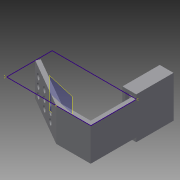
# Autodesk Inventor part: PiCamWalkerMount
Saved by Autodesk Inventor 2015 (Build 190159000, 159)
## iProperties
Created: 2016-04-28
Part Number: PiCamWalkerMount
Material: Generic
Document SubType Name: Modeling
Designer: Hatch
Density: 1 g/cm^3
Appearance: Default
Author: Hatch
Autodesk Inventor part; units mm, degrees
ref_plane "YZ Plane" through (0, 0, 0) normal (1, 0, 0) x (0, 1, 0)
ref_plane "XZ Plane" through (0, 0, 0) normal (0, 1, 0) x (-1, 0, 0)
ref_plane "XY Plane" through (0, 0, 0) normal (0, 0, 1) x (1, 0, 0)
sketch "Sketch1" plane through (0, 0, 0) normal (0, 1, 0) x (-1, 0, 0)
  line L0 (0, 0) -> (36, 0)
  line L1 (36, 0) -> (36, -24)
  line L2 (36, -24) -> (0, -24)
  line L3 (0, -24) -> (0, 0)
  dimension "d0" = 36
  dimension "d1" = 24
  constraints: 8 end point, 2 parallel, 1 horizontal, 1 perpendicular
  measures "d0" distance of L1.end L2.end
  measures "d1" distance of L0.end L1.end
extrude "Extrusion1" add sketch "Sketch1" along normal blind 3
sketch "Sketch2" plane through (0, 3, 0) normal (0, 1, 0) x (1, 0, 0)
  circle A0 centre (-6, 12) radius 2.125
  point P0 (0, 0)
  dimension "d4" = 4.25
  constraints: 1 centre point
  measures "d4" diameter of A0
extrude "Extrusion2" cut sketch "Sketch2" against normal through all
pattern_linear "Rectangular Pattern1" count 3 spacing 12 along (-1, 0, 0) count 3 spacing 6 along (0, 0, 1) of "Extrusion2" second direction both ways yes
sketch "Sketch3" plane through (0, 0, 0) normal (1, 0, 0) x (0, 0, -1)
  line L0 (0, 0) -> (24, 0)
  line L1 (24, 0) -> (24, 3)
  line L2 (24, 3) -> (0, 3)
  line L3 (0, 3) -> (0, 0)
  constraints: 8 end point, 2 parallel, 1 horizontal, 1 perpendicular
extrude "Extrusion3" add sketch "Sketch3" along normal blind 25
sketch "Sketch4" plane through (0, 3, 0) normal (0, 1, 0) x (1, 0, 0)
  line L0 (-36, 24) -> (25, 24) projected
  line L1 (25, 0) -> (22, 0)
  line L2 (22, 0) -> (22, 24)
  line L3 (22, 24) -> (25, 24)
  line L4 (25, 24) -> (25, 0)
  point P0 (0, 0)
  dimension "d15" = 3
  constraints: 8 end point, 2 parallel, 1 horizontal, 1 perpendicular, 1 point on line
  measures "d15" distance of L2.end L3.end
extrude "Extrusion4" add sketch "Sketch4" along normal blind 57
sketch "Sketch5" plane through (22, 3, -24) normal (-1, 0, 0) x (0, 0, 1)
  line L0 (24, 57) -> (24, 33)
  line L1 (24, -3) -> (24, 57) projected
  line L2 (0, -3) -> (0, 57) projected
  line L3 (24, 33) -> (0, 33)
  line L4 (0, 33) -> (0, 30)
  line L5 (0, 30) -> (24, 30)
  line L6 (24, 30) -> (24, 33)
  dimension "d18" = 24
  dimension "d19" = 3
  constraints: 10 end point, 2 parallel, 2 point on line, 1 horizontal, 1 perpendicular
  measures "d18" distance of L0.start L0.end
  measures "d19" distance of L4.end L3.end
extrude "Extrusion5" add sketch "Sketch5" along normal blind 7
sketch "Sketch6" plane through (22, 36, 0) normal (0, 1, 0) x (1, 0, 0)
  line L0 (-7, 0) -> (-5, 0)
  line L1 (-5, 0) -> (-5, 2)
  line L2 (-5, 2) -> (-7, 2)
  line L3 (-7, 2) -> (-7, 0)
  line L4 (-7, 24) -> (-5, 24)
  line L5 (-5, 24) -> (-5, 22)
  line L6 (-5, 22) -> (-7, 22)
  line L7 (-7, 22) -> (-7, 24)
  point P0 (-22, 0)
  dimension "d22" = 2
  dimension "d23" = 2
  dimension "d24" = 2
  dimension "d25" = 2
  constraints: 16 end point, 4 parallel, 2 horizontal, 2 perpendicular
  measures "d22" distance of L2.end L1.end
  measures "d23" distance of L1.end L0.end
  measures "d24" distance of L5.end L6.end
  measures "d25" distance of L4.end L5.end
extrude "Extrusion6" add sketch "Sketch6" along normal blind 24
sketch "Sketch7" plane through (25, 0, -24) normal (0, 0, -1) x (-1, 0, 0)
  line L0 (0, 60) -> (10, 60)
  line L1 (10, 60) -> (10, 33)
  line L2 (10, 33) -> (0, 33)
  line L3 (0, 33) -> (0, 60)
  point P0 (25, 0)
  constraints: 8 end point, 2 parallel, 1 horizontal, 1 perpendicular
extrude "Extrusion7" add sketch "Sketch7" along normal blind 3
sketch "Sketch8" plane through (-36, 0, 0) normal (0, 0, 1) x (1, 0, 0)
  line L0 (51, 33) -> (61, 33)
  line L1 (61, 33) -> (61, 60)
  line L2 (61, 60) -> (51, 60)
  line L3 (51, 60) -> (51, 33)
  point P0 (36, 0)
  constraints: 8 end point, 2 parallel, 1 horizontal, 1 perpendicular
extrude "Extrusion8" add sketch "Sketch8" along normal blind 3
sketch "Sketch9" plane through (-36, 0, 0) normal (0, 0, 1) x (1, 0, 0)
  line L0 (0, 0) -> (61, 0)
  line L1 (61, 0) -> (61, 33)
  line L2 (61, 33) -> (0, 33)
  line L3 (0, 33) -> (0, 0)
  point P0 (36, 0)
  constraints: 8 end point, 2 parallel, 1 horizontal, 1 perpendicular
sketch "Sketch10" plane through (0, 60, 0) normal (0, 1, 0) x (1, 0, 0)
  line L0 (22, 0) -> (22, -1)
  line L1 (22, 24) -> (22, 25)
  line L2 (22, -1) -> (17, -1)
  line L3 (17, -1) -> (17, 25)
  line L4 (17, 25) -> (22, 25)
  line L5 (22, 25) -> (22, -1)
  point P0 (0, 0)
  dimension "d34" = 1
  dimension "d35" = 1
  constraints: 12 end point, 2 parallel, 2 vertical, 1 horizontal, 1 perpendicular
  measures "d34" distance of L0.start L0.end
  measures "d35" distance of L1.start L1.end
extrude "Extrusion10" cut sketch "Sketch10" against normal through all
sketch "Sketch11" plane through (-36, 0, -24) normal (0, 0, -1) x (-1, 0, 0)
  line L0 (-58, 33) -> (-58, 0) projected
  line L1 (-53, 0) -> (-58, 0)
  line L2 (-58, 0) -> (-58, 3)
  line L3 (-58, 3) -> (-53, 3)
  line L4 (-53, 3) -> (-53, 0)
  point P0 (-36, 0)
  constraints: 8 end point, 2 parallel, 1 horizontal, 1 perpendicular, 1 point on line
extrude "Extrusion11" add sketch "Sketch11" against normal blind 24
sketch "Sketch12" plane through (-36, 0, -24) normal (0, 0, -1) x (-1, 0, 0)
  line L0 (-36, 0) -> (0, 20.7846)
  line L1 (-36, 0) -> (5.5692, 0) construction
  line L2 (0, 20.7846) -> (-1.5, 23.3827)
  line L3 (-1.5, 23.3827) -> (-37.5, 2.5981)
  line L4 (-37.5, 2.5981) -> (-36, 0)
  dimension "d47" = 30
  dimension "d48" = 3
  constraints: 10 end point, 2 perpendicular, 1 equal length, 1 horizontal
  measures "d47" angle of L1 L0
  measures "d48" distance of L0.end L2.end
ref_plane "Work Plane1" through (0.3404, 3, 0) normal (0.2240446, 0.9745789, 0) x (0.9745789, -0.2240446, 0)
extrude "Extrusion14" add sketch "Sketch12" against normal blind 24
sketch "Sketch15" plane through (-36, 0, -24) normal (0, 0, -1) x (-1, 0, 0)
  line L0 (0, 3) -> (-30.8038, 3)
  line L1 (0, 3) -> (-30.8038, 3) projected
  line L2 (-30.8038, 3) -> (-36, 0)
  line L3 (-36, 0) -> (0, 0)
  line L4 (0, 0) -> (-61, 0) projected
  line L5 (0, 0) -> (0, 3)
  constraints: 8 end point, 2 collinear, 1 perpendicular
extrude "Extrusion15" cut sketch "Sketch15" against normal through all
sketch "Sketch16" plane through (0.8038, 3, 0) normal (0.5, 0.8660254, 0) x (0.8660254, -0.5, 0)
  line L0 (-40.7654, 24) -> (-40.7654, 0) projected
  line L1 (-40.7654, 12) -> (-34.7654, 12)
  circle A0 centre (-34.7654, 12) radius 2.125
  point P0 (0.8038, 0)
  dimension "d53" = 6
  dimension "d54" = 4.25
  constraints: 2 end point, 1 centre point, 1 coincident, 1 horizontal, 1 midpoint
  measures "d53" distance of L1.start L1.end
  measures "d54" diameter of A0
extrude "Extrusion16" cut sketch "Sketch16" against normal through all
pattern_linear "Rectangular Pattern2" count 3 spacing 12 along (0.8660254, -0.5, 0) count 3 spacing 6 along (0, 0, 1) of "Extrusion16" second direction both ways yes
equation "\"d5\" = d4"
body "Solid1"
